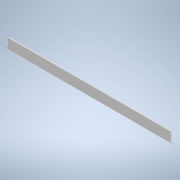
# Autodesk Inventor part: Acrylic Relief Guide
Saved by Autodesk Inventor 2020 (Build 240168000, 168)
## iProperties
Created: 2020-03-19
Part Number: Acrylic Relief Guide
Material: Generic
Document SubType Name: Modeling
Designer: DasNick
Density: 1 g/cm^3
Appearance: Default
Author: DasNick
Autodesk Inventor part; units mm, degrees
ref_plane "YZ Plane" through (0, 0, 0) normal (1, 0, 0) x (0, 1, 0)
ref_plane "XZ Plane" through (0, 0, 0) normal (0, 1, 0) x (-1, 0, 0)
ref_plane "XY Plane" through (0, 0, 0) normal (0, 0, 1) x (1, 0, 0)
sketch "Sketch1" plane through (0, 0, 0) normal (0, 0, 1) x (1, 0, 0)
  line L0 (34.925, -25.4) -> (34.925, 25.4) projected
  line L1 (34.925, 25.4) -> (-34.925, 25.4) projected
  line L2 (-34.925, 25.4) -> (-34.925, -25.4) projected
  line L3 (-34.925, -25.4) -> (34.925, -25.4) projected
  circle A0 centre (-30.1625, -16.6687) radius 2.3812 projected
  circle A1 centre (30.1625, -16.6688) radius 2.3812 projected
  circle A2 centre (30.1625, 15.0812) radius 2.3812 projected
  circle A3 centre (-30.1625, 15.0813) radius 2.3812 projected
  line L4 (771.525, -25.4) -> (771.525, 25.4) projected
  line L5 (771.525, 25.4) -> (701.675, 25.4) projected
  line L6 (701.675, 25.4) -> (701.675, -25.4) projected
  line L7 (701.675, -25.4) -> (771.525, -25.4) projected
  circle A4 centre (706.4375, -16.6688) radius 2.3812 projected
  circle A5 centre (766.7625, -16.6688) radius 2.3812 projected
  circle A6 centre (766.7625, 15.0812) radius 2.3812 projected
  circle A7 centre (706.4375, 15.0812) radius 2.3812 projected
  line L8 (34.925, -25.4) -> (701.675, -25.4)
  line L9 (701.675, 25.4) -> (34.925, 25.4)
  point P0 (0, 0)
  constraints: 4 end point, 1 parallel, 1 perpendicular
extrude "Extrusion1" add sketch "Sketch1" along normal blind 6.35
sketch "Sketch2" plane through (0, 0, 6.35) normal (0, 0, 1) x (1, 0, 0)
  line L0 (-34.925, 25.4) -> (-34.925, -25.4) projected
  line L1 (-34.925, 25.4) -> (-60.325, 25.4)
  line L2 (-60.325, 25.4) -> (-60.325, -25.4)
  line L3 (-60.325, -25.4) -> (-34.925, -25.4)
  line L4 (-34.925, -25.4) -> (-34.925, 25.4)
  circle A0 centre (-50.419, 12.7) radius 3.175
  circle A1 centre (-50.419, -12.7) radius 3.175
  point P0 (0, 0)
  dimension "d2" = 25.4
  dimension "d3" = 6.35
  dimension "d4" = 6.35
  dimension "d9" = 25.4
  dimension "d10" = 12.7
  constraints: 8 end point, 2 centre point
  measures "d2" distance of L0.start L1.end
  measures "d3" diameter of A0
  measures "d4" diameter of A1
  measures "d9" distance of A0.centre A1.centre
  measures "d10" distance from line of L1 A0.centre
extrude "Extrusion2" add sketch "Sketch2" against normal blind 6.35
body "Solid1"
